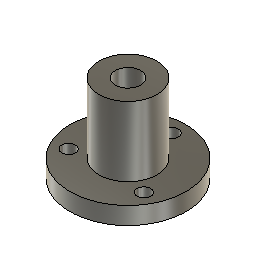
carridgedesignv24_FRAME DESIGN v14 (Autodesk Fusion 360 archive; units mm, degrees)
design "LSNUT"
Autodesk Fusion 360 part; units mm, degrees
sketch "Sketch1" plane through (0, 0, 0) normal (0, 0, 1) x (1, 0, 0)
  circle A0 centre (0, 0) radius 12.7
  circle A1 centre (0, 0) radius 2.7781
  dimension "d1" = 25.4
  dimension "d2" = 5.5563
  constraint coincident A0.centre A1.centre
  constraint concentric A0 A1
  measures "d1" diameter of A0
  measures "d2" diameter of A1
extrude "Extrude1" add sketch "Sketch1" along normal blind 3.81
sketch "Sketch2" plane through (0, 0, 3.81) normal (0, 0, 1) x (-1, 0, 0)
  circle A0 centre (0, 0) radius 2.7781
  circle A1 centre (0, 0) radius 12.7
  circle A2 centre (0, 0) radius 2.7781
  circle A3 centre (0, 0) radius 6.35
  line L0 (0, 0) -> (0, -12.7) construction
  line L1 (0, 0) -> (0, 12.7) construction
  line L2 (0, 0) -> (-12.7, 0) construction
  line L3 (0, 0) -> (12.7, 0) construction
  circle A4 centre (0, 0) radius 9.525 construction
  circle A5 centre (0, -9.525) radius 1.5
  arc A6 (-8.2489, 4.7625) -> (0, -9.525) centre (0, 0) ccw construction
  line L4 (0, 0) -> (-8.2489, 4.7625) construction
  line L5 (0, 0) -> (0, -9.525) construction
  arc A7 (0, -9.525) -> (8.2489, 4.7625) centre (0, 0) ccw construction
  line L6 (0, 0) -> (0, -9.525) construction
  line L7 (0, 0) -> (8.2489, 4.7625) construction
  circle A8 centre (-8.2489, 4.7625) radius 1.5
  circle A9 centre (8.2489, 4.7625) radius 1.5
  dimension "d5" = 5.5563
  dimension "d6" = 12.7
  dimension "d9" = 19.05
  dimension "d10" = 3
  dimension "d11" = 120
  dimension "d12" = 120
  dimension "d13" = 3
  dimension "d14" = 3
  constraint concentric A0 A2
  constraint concentric A2 A3
  constraint coincident A0.centre A1.centre
  constraint coincident A1 L0.end
  constraint vertical L0
  constraint coincident A1 L1.end
  constraint parallel L0 L1
  constraint coincident A1 L2.end
  constraint perpendicular L1 L2
  constraint coincident A1 L3.end
  constraint parallel L2 L3
  constraint coincident A4 A5.centre
  constraint coincident L0 A5.centre
  constraint coincident A5.centre A6.end
  constraint coincident A6.start L4.end
  constraint coincident A7.end L7.end
  measures "d5" diameter of A2
  measures "d6" diameter of A3
  measures "d9" diameter of A4
  measures "d10" diameter of A5
  measures "d11" angle of L4 L5
  measures "d12" angle of L6 L7
  measures "d13" diameter of A8
  measures "d14" diameter of A9
extrude "Extrude3" cut sketch "Sketch2" against normal blind 3.81 contours A5 | A8 | A9
extrude "Extrude2" add sketch "Sketch2" along normal blind 15.24 contours A3
equation "d7 = 19.05 mm - 3.81 mm"
